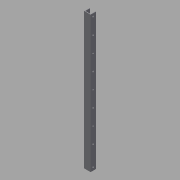
# Autodesk Inventor part: 26in C-Channel
Saved by Autodesk Inventor 2013 (Build 170138000, 138)
## iProperties
Created: 2013-01-08
Part Number: 26in C-Channel
Material: Generic
Document SubType Name: Modeling
Designer: Naphat
Density: 1 g/cm^3
Author: Naphat
Autodesk Inventor part; units mm, degrees
ref_plane "YZ Plane" through (0, 0, 0) normal (1, 0, 0) x (0, 1, 0)
ref_plane "XZ Plane" through (0, 0, 0) normal (0, 1, 0) x (-1, 0, 0)
ref_plane "XY Plane" through (0, 0, 0) normal (0, 0, 1) x (1, 0, 0)
sketch "Sketch1" plane through (0, 0, 0) normal (0, 0, 1) x (1, 0, 0)
  line L0 (-15.7, 12.7) -> (-12.7, 12.7)
  line L1 (-12.7, 12.7) -> (-12.7, -9.7)
  line L2 (-12.7, -9.7) -> (12.7, -9.7)
  line L3 (12.7, -9.7) -> (12.7, 12.7)
  line L4 (12.7, 12.7) -> (15.7, 12.7)
  line L5 (15.7, 12.7) -> (15.7, -12.7)
  line L6 (15.7, -12.7) -> (-15.7, -12.7)
  line L7 (-15.7, -12.7) -> (-15.7, 12.7)
  point P0 (0, 0)
  dimension "d0" = 3
  dimension "d2" = 3
  dimension "d3" = 25.4
  dimension "d4" = 31.4
  dimension "d5" = 15.7
  dimension "d7" = 12.7
  dimension "d8" = 3
  constraints: 16 end point, 5 parallel, 1 collinear, 1 horizontal, 1 perpendicular
  measures "d0" distance of L0.start L0.end
  measures "d2" distance of L3.end L4.end
  measures "d3" distance of L6.end L0.start
  measures "d4" distance of L5.end L6.end
  measures "d5" distance from line of point (0, 0) L7
  measures "d7" distance from line of L6 point (0, 0)
  measures "d8" distance between parallel lines of L6 L2
extrude "Extrusion1" add sketch "Sketch1" against normal blind 660.4
sketch "Sketch5" plane through (15.7, -12.7, 0) normal (1, 0, 0) x (0, 0, -1)
  circle A0 centre (13.8784, 12.3) radius 3.175
  circle A1 centre (91.9, 12.3) radius 3.175
  circle A2 centre (168.1, 12.3) radius 3.175
  circle A3 centre (244.3, 12.3) radius 3.175
  circle A4 centre (320.5, 12.3) radius 3.175
  circle A5 centre (396.7, 12.3) radius 3.175
  circle A6 centre (472.9, 12.3) radius 3.175
  circle A7 centre (549.1, 12.3) radius 3.175
  circle A8 centre (645.6513, 12.3) radius 3.175
  point P0 (0, 12.7)
  dimension "d56" = 6.35
  dimension "d58" = 6.35
  dimension "d59" = 6.35
  dimension "d60" = 6.35
  dimension "d61" = 6.35
  dimension "d62" = 6.35
  dimension "d63" = 6.35
  dimension "d64" = 6.35
  dimension "d65" = 6.35
  constraints: 9 centre point
  measures "d56" diameter of A0
  measures "d58" diameter of A1
  measures "d59" diameter of A2
  measures "d60" diameter of A3
  measures "d61" diameter of A4
  measures "d62" diameter of A5
  measures "d63" diameter of A6
  measures "d64" diameter of A7
  measures "d65" diameter of A8
extrude "Extrusion5" cut sketch "Sketch5" against normal blind 76.2
equation "\"d2\" = d0"
equation "\"d5\" = 0.5 * d4"
equation "\"d7\" = 0.5 * d3"
equation "\"d8\" = d0"
equation "\"d58\" = d56"
equation "\"d59\" = d58"
equation "\"d60\" = d59"
equation "\"d61\" = d60"
equation "\"d62\" = d61"
equation "\"d63\" = d62"
equation "\"d64\" = d63"
equation "\"d65\" = d64"
body "Solid1"
